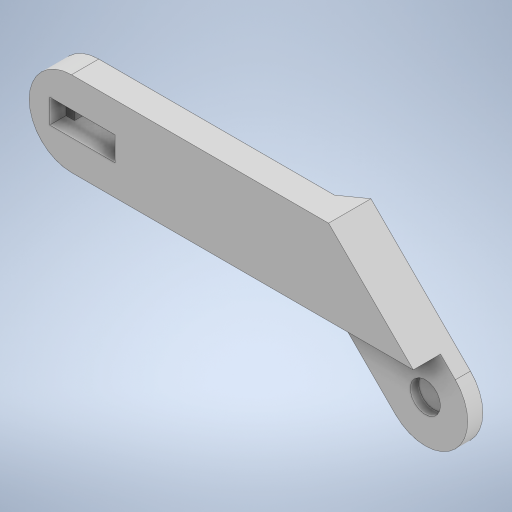
# Autodesk Inventor part: arm 1 right
Saved by Autodesk Inventor 2023 (Build 270158000, 158)
## iProperties
Created: 2024-06-28
Part Number: arm 1 right
Material: Generic
Document SubType Name: Modeling
Designer: Swoby
Density: 1 g/cm^3
Appearance: Default
Author: Swoby
Autodesk Inventor part; units mm, degrees
ref_plane "YZ Plane" through (0, 0, 0) normal (1, 0, 0) x (0, 1, 0)
ref_plane "XZ Plane" through (0, 0, 0) normal (0, 1, 0) x (-1, 0, 0)
ref_plane "XY Plane" through (0, 0, 0) normal (0, 0, 1) x (1, 0, 0)
sketch "Sketch1" plane through (0, 0, 0) normal (0, 0, 1) x (1, 0, 0)
  circle A0 centre (0, 0) radius 35
  circle A1 centre (270, -72) radius 35
  line L0 (0, 35) -> (212.4975, 35)
  line L1 (212.4975, 35) -> (294.7487, -47.2513)
  line L2 (0, -35) -> (183.5025, -35)
  line L3 (183.5025, -35) -> (245.2513, -96.7487)
  dimension "d0" = 70
  dimension "d1" = 70
  dimension "d2" = 135
  dimension "d3" = 37
  dimension "d4" = 270
  constraints: 8 end point, 4 point on circle, 4 tangent, 2 centre point, 2 parallel, 1 coincident, 1 horizontal
  measures "d0" diameter of A0
  measures "d1" diameter of A1
  measures "d2" angle of L1 L0
  measures "d3" distance from line of L2 A1.centre
  measures "d4" horizontal distance of A1.centre point (0, 0)
extrude "Extrusion1" add sketch "Sketch1" along normal blind 22.5
sketch "Sketch2" plane through (0, 0, 22.5) normal (0, 0, 1) x (1, 0, 0)
  circle A0 centre (0, 0) radius 2.5
  line L0 (-18, 10) -> (29, 10)
  line L1 (29, 10) -> (29, -10)
  line L2 (29, -10) -> (-18, -10)
  line L3 (-18, -10) -> (-18, 10)
  line L4 (-11, 10) -> (36, 10)
  line L5 (36, 10) -> (36, -10)
  line L6 (36, -10) -> (-11, -10)
  line L7 (-11, -10) -> (-11, 10)
  line L8 (-18, 0) -> (36, 0) construction
  point P0 (29, 10)
  dimension "d7" = 5
  dimension "d9" = 54
  dimension "d10" = 40
  dimension "d11" = 7
  dimension "d12" = 36
  dimension "d13" = 20
  constraints: 18 end point, 4 parallel, 3 point on line, 2 horizontal, 2 midpoint, 2 perpendicular, 1 centre point, 1 coincident
  measures "d7" diameter of A0
  measures "d9" distance of L4.end L0.start
  measures "d10" distance between parallel lines of L1 L7
  measures "d11" distance between parallel lines of L3 L7
  measures "d12" distance from line of point (0, 0) L5
  measures "d13" distance of L4.end L5.end
extrude "Extrusion2" cut sketch "Sketch2" against normal through all contours A0 | L0 L1 L2 L7
extrude "Extrusion3" cut sketch "Sketch2" against normal blind 13.5 contours L0 L7 L2 L3 | L4 L5 L6 L1
sketch "Sketch3" plane through (0, 0, 0) normal (0, 0, -1) x (-1, 0, 0)
  arc A0 (-294.7487, -47.2513) -> (-245.2513, -96.7487) centre (-270, -72) ccw projected
  line L0 (-183.5025, -35) -> (-245.2513, -96.7487) projected
  line L1 (0, -35) -> (-183.5025, -35) projected
  arc A1 (0, -35) -> (0, 35) centre (0, 0) ccw projected
  line L2 (-212.4975, 35) -> (0, 35) projected
  line L3 (-294.7487, -47.2513) -> (-212.4975, 35) projected
  line L4 (0, -35) -> (-183.5025, -35) projected
  line L5 (-212.4975, 35) -> (-142.4975, -35)
  point P0 (-142.4975, -35)
  dimension "d18" = 135
  constraints: 2 end point, 1 point on line
  measures "d18" angle of L1 L5
extrude "Extrusion4" add sketch "Sketch3" along normal blind 12.5 contours L3 L5 L1 L0 A0
chamfer "Chamfer1" distance 12.5 angle 45 1 edges at (177.4975, 0, 0)
sketch "Sketch4" plane through (0, 0, 22.5) normal (0, 0, 1) x (1, 0, 0)
  line L0 (183.5025, -35) -> (245.2513, -96.7487) projected
  arc A0 (245.2513, -96.7487) -> (294.7487, -47.2513) centre (270, -72) ccw projected
  line L1 (294.7487, -47.2513) -> (212.4975, 35) projected
  line L2 (212.4975, 35) -> (0, 35) projected
  arc A1 (0, 35) -> (0, -35) centre (0, 0) ccw projected
  line L3 (0, -35) -> (183.5025, -35) projected
  line L4 (183.5025, -35) -> (245.2513, -96.7487) projected
  line L5 (-18, 10) -> (36, 10) projected
  line L6 (36, 10) -> (36, -10) projected
  line L7 (36, -10) -> (-18, -10) projected
  line L8 (-18, -10) -> (-18, 10) projected
  line L9 (245.2513, -96.7487) -> (183.5025, -35) projected
  line L10 (183.5025, -35) -> (282.4975, -35)
  constraints: 2 end point, 1 horizontal, 1 point on line
extrude "Extrusion5" cut sketch "Sketch4" against normal blind 22.5 contours L10 L1 A0 L0
sketch "Sketch5" plane through (0, 0, 0) normal (0, 0, 1) x (1, 0, 0)
  arc A0 (245.2513, -96.7487) -> (294.7487, -47.2513) centre (270, -72) ccw projected
  circle A1 centre (270, -72) radius 12.5
  point P0 (0, 0)
  dimension "d26" = 25
  constraints: 1 centre point, 1 coincident
  measures "d26" diameter of A1
extrude "Extrusion6" cut sketch "Sketch5" against normal blind 7
body "Solid1"
